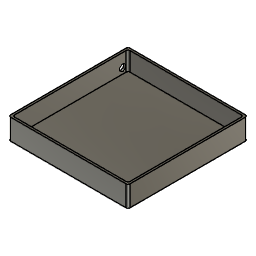
Case (Autodesk Fusion 360 design; units mm, degrees)
Autodesk Fusion 360 part; units mm, degrees
sketch "Esboço1" plane through (0, 0, 0) normal (0, 0, 1) x (1, 0, 0) in component "CASE"
  line L0 (-57.5, 57.5) -> (57.5, 57.5)
  line L1 (57.5, 57.5) -> (57.5, -57.5)
  line L2 (57.5, -57.5) -> (-57.5, -57.5)
  line L3 (-57.5, -57.5) -> (-57.5, 57.5)
  line L4 (-57.5, 57.5) -> (57.5, -57.5) construction
  line L5 (57.5, 57.5) -> (-57.5, -57.5) construction
  dimension "d5" = 115
  dimension "d6" = 115
  constraint horizontal L0
  constraint perpendicular L0 L1
  constraint parallel L0 L2
  constraint parallel L1 L3
  constraint coincident L4 origin
  constraint coincident L5 origin
  measures "d5" distance of L1.end L2.end
  measures "d6" distance of L0.end L1.end
sketch "Esboço2" plane through (0, 0, 0) normal (1, 0, 0) x (0, 1, 0) in component "CASE"
extrude "Extrusão1" add sketch "Esboço1" along normal blind 20 in component "CASE"
fillet "Arredondamento1" radius 4 4 edges at (57.5, -57.5, 10) (57.5, 57.5, 10) (-57.5, 57.5, 10) (-57.5, -57.5, 10) in component "CASE"
shell "Casca1" thickness 2 removed faces 1 at (-17.8333, -16.5, 20) in component "CASE"
delete_face "Excluir face1" 1 faces at (-55.3329, 57.0553, 6.6667) in component "CASE"
hole "Furo1" at (-57.5, 50.4054, 7.3062) direction (1, 0, 0) diameter 6 depth 4 tip angle 118 in component "CASE"
fillet "Arredondamento2" radius 2 1 edges at (-57.5, 57.5, 10) in component "CASE"
delete_face "Excluir face2" 1 faces at (-57.4955, -53.6903, 6.6667) in component "CASE"
fillet "Arredondamento3" radius 2 1 edges at (-57.5, -57.5, 10) in component "CASE"
delete_face "Excluir face3" 1 faces at (53.6903, -57.4955, 6.6667) in component "CASE"
fillet "Arredondamento4" radius 2 1 edges at (57.5, -57.5, 10) in component "CASE"
delete_face "Excluir face4" 1 faces at (55.3329, 57.0553, 6.6667) in component "CASE"
fillet "Arredondamento5" radius 2 1 edges at (57.5, 57.5, 10) in component "CASE"
component "CASE" placed x (1, 0, 0) y (0, 1, 0) z (0, 0, 1) at (0, 0, 0)
equation "COMPRIMENTO = 115 mm"
equation "ALTURA = 20 mm"
equation "SHELL = 2 mm"
equation "GAP = 0.2 mm"
equation "d5 = COMPRIMENTO"
equation "d6 = COMPRIMENTO"
equation "d7 = ALTURA"
equation "d11 = SHELL"
